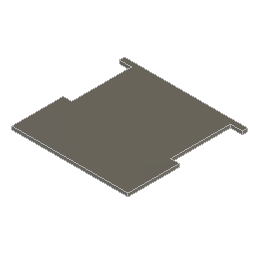
Spool Stand (Autodesk Fusion 360 archive; units mm, degrees)
design "Flaps"
part number: 2026-02-24-16-08-38-778
Autodesk Fusion 360 part; units mm, degrees
sketch "Sketch1" plane through (0, 0, 0) normal (0, 0, 1) x (1, 0, 0)
  line L0 (24, 9.5) -> (24, -22)
  line L1 (23, -23) -> (-9, -23)
  line L2 (-10, -22) -> (-10, 9.5)
  line L3 (-11, 11) -> (25, 11)
  line L4 (25, 11) -> (25, 9.5)
  line L5 (-11, 9.5) -> (-11, 11)
  line L6 (-11, 9.5) -> (-10, 9.5)
  line L7 (24, 9.5) -> (25, 9.5)
  line L8 (-10, -22) -> (-10, -23)
  line L9 (-10, -23) -> (-9, -23)
  line L10 (23, -23) -> (24, -23)
  line L11 (24, -23) -> (24, -22)
  point P0 (24, -23)
  point P1 (-10, -23)
  dimension "d3" = 1.5
  dimension "d4" = 34
  dimension "d5" = 1
  dimension "d6" = 34
  constraint vertical L0
  constraint horizontal L1
  constraint vertical L2
  constraint horizontal L3
  constraint vertical L4
  constraint vertical L5
  constraint coincident P1 L1
  constraint coincident P1 L2
  constraint coincident P0 L0
  constraint coincident P0 L1
  constraint perpendicular L2 L6
  constraint perpendicular L4 L7
  constraint coincident P1 L8.end
  constraint coincident P0 L10.end
  measures "d3" distance of L3.end L4.end
  measures "d4" vertical distance of P1 L3.start
  measures "d5" distance of L2.end L5.start
  measures "d6" distance of P0 P1
extrude "Extrude3" add sketch "Sketch1" along normal blind 2
sketch "Sketch7" plane through (0, 0, 2) normal (0, 0, 1) x (-1, 0, 0)
  line L0 (10, 23) -> (-24, 23)
  line L1 (-24, 23) -> (-24, -9.5)
  line L2 (-24, -9.5) -> (-25, -9.5)
  line L3 (-25, -9.5) -> (-25, -11)
  line L4 (-25, -11) -> (11, -11)
  line L5 (11, -11) -> (11, -9.5)
  line L6 (11, -9.5) -> (10, -9.5)
  line L7 (10, -9.5) -> (10, 23)
  line L8 (10, -9.5) -> (7.5, -9.5)
  line L9 (7.5, -9.5) -> (7.5, 8)
  line L10 (7.5, 8) -> (10, 8)
  line L11 (10, 8) -> (10, -9.5)
  line L12 (-24, -9.5) -> (-21.5, -9.5)
  line L13 (-21.5, -9.5) -> (-21.5, 8)
  line L14 (-21.5, 8) -> (-24, 8)
  line L15 (-24, 8) -> (-24, -9.5)
  dimension "d26" = 2.5
  dimension "d27" = 2.5
  constraint horizontal L8
  constraint vertical L9
  constraint horizontal L10
  constraint vertical L11
  constraint coincident L6.end L7.start
  constraint horizontal L12
  constraint vertical L13
  constraint horizontal L14
  constraint vertical L15
  constraint coincident L1.end L2.start
  measures "d26" distance of L6.end L8.end
  measures "d27" distance of L1.end L12.end
extrude "Extrude4" cut sketch "Sketch7" against normal blind 2 contours L7 L8 L9 L10 L11 | L1 L12 L13 L14 L15
extrude "Extrude5" cut 1 faces at (2.1667, 3.6667, 2) along direction (0, 0, -1) blind 1
